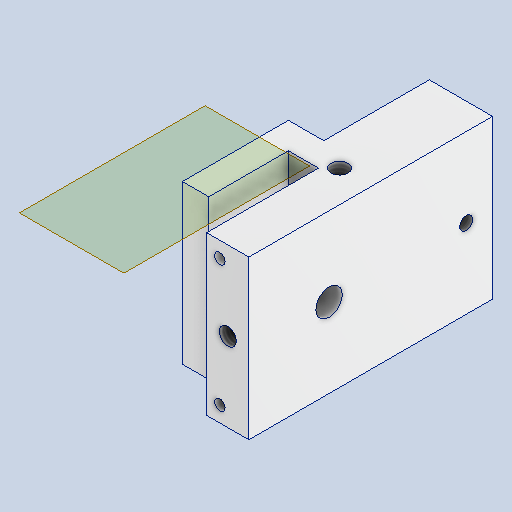
# Autodesk Inventor part: Katze_Lagerhalter_vorne
Saved by Autodesk Inventor 2025 (Build 290162010, 162A)
## iProperties
Created: 2024-11-12
Part Number: Katze_Lagerhalter_vorne
Material: Aluminium 6061, Katze
Document SubType Name: Modeling
Designer: Admin
Density: 2.7 g/cm^3
Appearance: Aluminium - flach(1)
Author: Admin
Autodesk Inventor part; units mm, degrees
ref_plane "YZ Plane" through (0, 0, 0) normal (1, 0, 0) x (0, 1, 0)
ref_plane "XZ Plane" through (0, 0, 0) normal (0, 1, 0) x (-1, 0, 0)
ref_plane "XY Plane" through (0, 0, 0) normal (0, 0, 1) x (1, 0, 0)
ref_plane "Arbeitsebene1" through (0, 0, 0) normal (0, 0, -1) x (-1, 0, 0)
sketch "Skizze1" plane through (0, 0, 0) normal (0, 0, -1) x (-1, 0, 0)
  line L0 (-9, -16) -> (-9, 16) construction
  line L1 (-9, 16) -> (-7.5, 16) construction
  line L2 (-7.5, -1) -> (-7.5, -16) construction
  line L3 (-11.1, -3.1) -> (-19.1, -3.1) construction
  line L4 (-19.1, -3.1) -> (-19.1, 43.1)
  line L5 (-19.1, 43.1) -> (-7.1, 43.1)
  line L6 (-7.1, 23.1) -> (-0.4, 23.1)
  line L7 (-0.4, 23.1) -> (-0.4, 3)
  line L8 (-0.4, 3) -> (-5.4, 3)
  line L9 (-5.4, 3) -> (-5.4, 18.1)
  line L10 (-5.4, 18.1) -> (-11.1, 18.1)
  line L11 (-11.1, 18.1) -> (-11.1, -3.1)
  line L12 (-19.1, -3.1) -> (-11.1, -3.1)
  line L13 (-11.1, -3.1) -> (-9, -3.1) construction
  line L14 (-9, 18.1) -> (-9, 16) construction
  line L15 (-7.5, 16) -> (-5.4, 16) construction
  line L16 (-7.1, 23.1) -> (-7.1, 43.1)
  point P0 (0, 0)
  dimension "d0" = 20
  dimension "d1" = 5
  dimension "d2" = 5
  dimension "d3" = 13
  dimension "d18" = 12
  constraints: 26 end point, 9 perpendicular, 4 point on line, 2 equal length, 2 vertical, 1 collinear, 1 parallel
  measures "d0" distance from line of L6.start L5
  measures "d1" distance between parallel lines of L10 L6
  measures "d2" distance between parallel lines of L9 L7
  measures "d3" distance from line of L8 L15.end
  measures "d18" distance between parallel lines of L4 L16
extrude "Extrusion1" add sketch "Skizze1" along normal blind 30
sketch "Skizze2" plane through (7.1, 23.1, 0) normal (-1, 0, 0) x (0, 0, 1)
  line L0 (0, 20) -> (-30, 20) projected
  line L1 (-15, 15) -> (-15, 20) construction
  point P0 (0, -23.1)
  point P1 (-15, 20)
  point P2 (-15, 20)
  dimension "d6" = 5
  constraints: 4 midpoint, 2 end point, 1 coincident, 1 perpendicular, 1 point on line
  measures "d6" distance of L1.start L1.end
hole "gewindeLastPunkt" at (7.1, 38.1, -15) direction (1, 0, 0) diameter 2.459 end through all thread size "M3x0.5" class "6H" standard "ANSI Metric M Profile"
sketch "Skizze3" plane through (11.1, -3.1, 0) normal (0, -1, 0) x (1, 0, 0)
  circle A0 centre (4, -15) radius 2 construction
  point P0 (-11.1, 0)
  constraints: 1 coincident
hole "Katzeverbindung" at (15.1, -3.1, -15) direction (0, 1, 0) diameter 3.242 depth 11.8 tip angle 118 thread size "M4x0.7" class "6H" standard "ANSI Metric M Profile"
sketch "Skizze4" plane through (11.1, -3.1, 0) normal (0, -1, 0) x (1, 0, 0)
  circle A0 centre (2.5, -27) radius 1 projected
  circle A1 centre (2.5, -3) radius 1 projected
  point P0 (-11.1, 0)
hole "Zentrierbolzen" at (13.6, -3.1, -3) at (13.6, -3.1, -27) direction (0, 1, 0) diameter 2 depth 6 tip angle 118
sketch "Skizze5" plane through (0, 0, 0) normal (0, 0, 1) x (1, 0, 0)
  line L0 (19.1, 43.1) -> (19.1, -3.1) projected
  line L1 (7.1, 43.1) -> (19.1, 43.1) projected
  point P0 (0, 0)
  point P1 (13.1, 20.1)
  dimension "d92" = 6
  dimension "d93" = 23
  measures "d92" distance from line of L0 point (13.1, 20.1)
  measures "d93" distance from line of L1 point (13.1, 20.1)
hole "seilV" at (13.1, 20.1, 0) direction (0, 0, -1) diameter 3.242 end through all thread size "M4x0.7" class "6H" standard "ANSI Metric M Profile"
sketch "Skizze6" plane through (5.4, 18.1, 0) normal (0, -1, 0) x (1, 0, 0)
  line L0 (5.7, 0) -> (0, 0) construction
  line L1 (0, 0) -> (0, -30) construction
  line L2 (5.7, -30) -> (0, -30) construction
  line L3 (5.7, 0) -> (5.7, -30) construction
  line L4 (5.7, -15) -> (2.85, -15) construction
  line L5 (2.85, -15) -> (2.85, -30) construction
  line L6 (2.85, -15) -> (2.85, 0) construction
  line L7 (2.85, -15) -> (0, -15) construction
  line L8 (5.7, 0) -> (5.7, -30) construction
  point P0 (-5.4, 0)
  constraints: 8 end point, 4 midpoint, 1 horizontal, 1 parallel
hole "GLVV" at (8.25, 18.1, -15) direction (0, 1, 0) diameter 1.567 depth 4 tip angle 118 thread size "M2x0.4" class "6H" standard "ANSI Metric M Profile"
sketch "Skizze7" plane through (11.1, -3.1, 0) normal (-1, 0, 0) x (0, 0, 1)
  line L0 (-30, 19.2) -> (0, 19.2) construction
  line L1 (0, 0) -> (0, 21.2) construction
  line L2 (0, 21.2) -> (-30, 21.2) construction
  line L3 (-30, 0) -> (-30, 21.2) construction
  line L4 (0, 0) -> (-30, 0) construction
  line L5 (-30, 10.2) -> (-15, 10.2) construction
  line L6 (-15, 10.2) -> (0, 10.2) construction
  line L7 (-15, 10.2) -> (-15, 19.2) construction
  point P0 (0, 3.1)
  dimension "d62" = 9
  constraints: 6 end point, 3 point on line, 1 collinear, 1 horizontal, 1 midpoint, 1 perpendicular
  measures "d62" distance of L5.end L7.end
hole "GLVO" at (11.1, 7.1, -15) direction (1, 0, 0) diameter 1.567 depth 4 tip angle 118 thread size "M2x0.4" class "6H" standard "ANSI Metric M Profile"
sketch "Skizze8" plane through (5.4, 3, 0) normal (1, 0, 0) x (0, 0, -1)
  line L0 (0, 15.1) -> (0, 0) construction
  line L1 (0, 0) -> (30, 0) construction
  line L2 (30, 15.1) -> (30, 0) construction
  line L3 (0, 15.1) -> (30, 15.1) construction
  line L4 (0, 13.1) -> (30, 13.1) construction
  line L5 (15, 9.1) -> (15, 13.1) construction
  line L6 (15, 9.1) -> (0, 9.1) construction
  line L7 (15, 9.1) -> (30, 9.1) construction
  line L8 (30, 15.1) -> (30, 0) construction
  point P0 (0, -3)
  dimension "d70" = 4
  constraints: 6 end point, 3 point on line, 2 perpendicular, 1 collinear, 1 midpoint
  measures "d70" distance of L5.start L5.end
hole "GLVU" at (5.4, 12.1, -15) direction (-1, 0, 0) diameter 1.567 depth 4 tip angle 118 thread size "M2x0.4" class "6H" standard "ANSI Metric M Profile"
sketch "Skizze9" plane through (0.4, 3, 0) normal (-1, 0, 0) x (0, 0, 1)
  circle A0 centre (-15, 4.1) radius 1 projected
  point P0 (0, -3)
hole "DLVU" at (0.4, 7.1, -15) direction (1, 0, 0) diameter 5 depth 5
sketch "Skizze10" plane through (11.1, -3.1, 0) normal (-1, 0, 0) x (0, 0, 1)
  circle A0 centre (-15, 15.2) radius 0.7835 projected
  point P0 (0, 3.1)
hole "DLVO" at (11.1, 12.1, -15) direction (1, 0, 0) diameter 5 end through all
